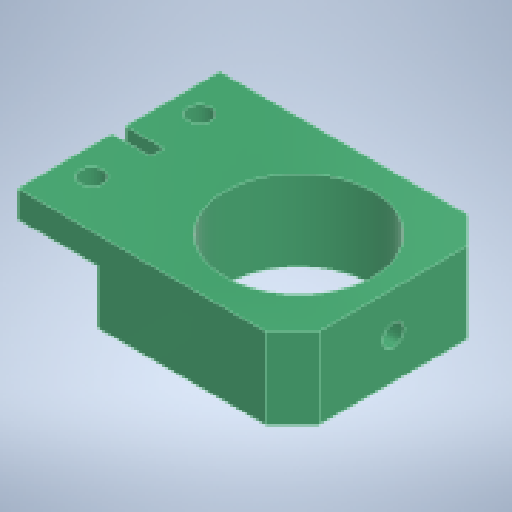
# Autodesk Inventor part: креп_маркера
Saved by Autodesk Inventor 2023.1 (Build 271208000, 208)
## iProperties
Created: 2026-01-10
Part Number: креп_маркера
Material: Полипропилен
Document SubType Name: Modeling
Designer: DELL
Density: 0.899 g/cm^3
Appearance: Гладкий — темный цвет морской волны
Author: DELL
Autodesk Inventor part; units mm, degrees
ref_plane "YZ Plane" through (0, 0, 0) normal (1, 0, 0) x (0, 1, 0)
ref_plane "XZ Plane" through (0, 0, 0) normal (0, 1, 0) x (-1, 0, 0)
ref_plane "XY Plane" through (0, 0, 0) normal (0, 0, 1) x (1, 0, 0)
sketch "Эскиз1" plane through (0, 0, 0) normal (0, 1, 0) x (-1, 0, 0)
  line L0 (0, 15) -> (10, 15)
  line L1 (10, 15) -> (10, -15)
  line L2 (10, -15) -> (0, -15)
  line L3 (0, -15) -> (0, 15)
  circle A0 centre (11.75, 8) radius 1.75
  circle A1 centre (11.75, -8) radius 1.75
  line L4 (15.75, 15) -> (7.75, 15)
  line L5 (7.75, 15) -> (7.75, 1)
  line L6 (7.75, 1) -> (15.75, 1)
  line L7 (15.75, 1) -> (15.75, 15)
  line L8 (15.75, 15) -> (7.75, 1) construction
  line L9 (7.75, 15) -> (15.75, 1) construction
  line L10 (15.75, -1) -> (7.75, -1)
  line L11 (7.75, -1) -> (7.75, -15)
  line L12 (7.75, -15) -> (15.75, -15)
  line L13 (15.75, -15) -> (15.75, -1)
  line L14 (15.75, -1) -> (7.75, -15) construction
  line L15 (7.75, -1) -> (15.75, -15) construction
  point P0 (0, 0)
  point P1 (10, -1)
  point P2 (10, 1)
  point P3 (10, 15)
  point P4 (0, 0)
  dimension "d0" = 10
  dimension "d1" = 30
  dimension "d2" = 3.5
  dimension "d3" = 3.5
  dimension "d4" = 7
  dimension "d5" = 7
  dimension "d6" = 4
  dimension "d7" = 4
  constraints: 32 end point, 6 parallel, 5 midpoint, 3 horizontal, 3 perpendicular, 2 centre point, 2 point on line, 2 tangent, 1 coincident
  measures "d0" distance of L1.end L2.end
  measures "d1" distance of L0.end L1.end
  measures "d2" diameter of A0
  measures "d3" diameter of A1
  measures "d4" distance from line of A0.centre L0
  measures "d5" distance from line of A1.centre L2
  measures "d6" distance from line of L7 A0.centre
  measures "d7" distance from line of L13 A1.centre
extrude "Выдавливание1" add sketch "Эскиз1" along normal blind 4
sketch "Эскиз2" plane through (0, 0, 0) normal (0, -1, 0) x (1, 0, 0)
  line L0 (-15.75, 15) -> (0, 15) projected
  line L1 (0, -15) -> (-15.75, -15) projected
  line L2 (0, 15) -> (-4, 15)
  line L3 (-4, 15) -> (-4, -15)
  line L4 (-4, -15) -> (0, -15)
  line L5 (0, -15) -> (0, 15)
  line L6 (-10, -1) -> (-10, 1) projected
  line L7 (-10, 1) -> (-10, 15) construction
  line L8 (-15.75, 15) -> (0, 15) projected
  point P0 (0, 0)
  point P1 (-4, 15)
  point P2 (-10, 0)
  dimension "d27" = 6
  constraints: 10 end point, 2 parallel, 2 point on line, 1 horizontal, 1 midpoint, 1 perpendicular, 1 vertical
  measures "d27" distance from line of point (-10, 0) L3
extrude "Выдавливание2" add sketch "Эскиз2" along normal blind 8
sketch "Эскиз3" plane through (0, 4, 0) normal (0, 1, 0) x (1, 0, 0)
  circle A0 centre (11, 0) radius 11
  line L0 (-15.75, -15) -> (0, -15) projected
  line L1 (0, -15) -> (25, -15)
  line L2 (0, -15) -> (0, 15)
  line L3 (0, 15) -> (-15.75, 15) projected
  line L4 (0, 15) -> (25, 15)
  line L5 (25, 15) -> (25, -15)
  point P0 (0, 0)
  dimension "d13" = 22
  dimension "d14" = 11
  dimension "d15" = 14
  constraints: 8 end point, 2 point on line, 1 centre point, 1 collinear, 1 horizontal, 1 perpendicular, 1 vertical
  measures "d13" diameter of A0
  measures "d14" distance of point (0, 0) A0.centre
  measures "d15" distance from line of L5 A0.centre
extrude "Выдавливание3" add sketch "Эскиз3" against normal up to surface (12 mm away)
sketch "Эскиз4" plane through (25, 4, 15) normal (1, 0, 0) x (0, 0, -1)
  line L0 (0, 0) -> (0, -12) construction
  line L1 (30, 0) -> (30, -12) construction
  line L2 (30, -4) -> (30, 0) construction
  line L3 (30, 0) -> (0, -12) construction
  circle A0 centre (15, -6) radius 1.6
  dimension "d19" = 3.2
  constraints: 2 end point, 1 centre point, 1 midpoint
  measures "d19" diameter of A0
extrude "Выдавливание4" cut sketch "Эскиз4" against normal blind 10
chamfer "Фаска1" distance 4 angle 45 2 edges at (25, -2, 15) (25, -2, -15)
